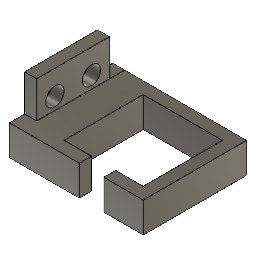
holder_R v6 (Autodesk Fusion 360 design; units mm, degrees)
Autodesk Fusion 360 part; units mm, degrees
sketch "Sketch1" plane through (0, 0, 0) normal (0, 0, 1) x (1, 0, 0)
  line L0 (0, 0) -> (13, 0)
  line L1 (13, 0) -> (13, 13)
  line L2 (13, 13) -> (0, 13)
  line L3 (0, 13) -> (0, 0)
  line L4 (-2, -2) -> (15, -2)
  line L5 (15, -2) -> (15, 15)
  line L6 (15, 15) -> (-2, 15)
  line L7 (-2, 15) -> (-2, -2)
  dimension "d1" = 13
  dimension "d2" = 13
  dimension "d3" = 2
  constraint horizontal L0
  constraint vertical L1
  constraint horizontal L2
  constraint vertical L3
  constraint coincident L0.start L3.end
  measures "d1" distance of L1.end L2.end
  measures "d2" distance of L0.end L1.end
extrude "Extrude1" add sketch "Sketch1" along normal blind 5
sketch "Sketch2" plane through (0, 0, 0) normal (0, 1, 0) x (-1, 0, 0)
  line L0 (-13, 0) -> (0, 0)
  line L1 (0, 0) -> (0, 5)
  line L2 (0, 5) -> (-13, 5)
  line L3 (-13, 5) -> (-13, 0)
  line L4 (-8.5, 5) -> (-4.5, 5)
  line L5 (-4.5, 5) -> (-4.5, 0)
  line L6 (-4.5, 0) -> (-8.5, 0)
  line L7 (-8.5, 0) -> (-8.5, 5)
  line L8 (-6.5, 0) -> (-6.5, 5)
  dimension "d6" = 4
  dimension "d7" = 90
  constraint horizontal L4
  constraint vertical L5
  constraint horizontal L6
  constraint vertical L7
  constraint coincident L0 L5.end
  constraint coincident L2 L4.start
  constraint midpoint L6 L8.start
  constraint midpoint L2 L8.end
  measures "d6" distance of L4.start L4.end
  measures "d7" angle of L4 L8
extrude "Extrude2" cut sketch "Sketch2" against normal blind 10 contours L0 L2 L4 L6 L7 L8 | L0 L2 L4 L5 L6 L8
extrude "Extrude3" add 1 faces at (-2, 9.3333, 1.6667) along direction (-1, 0, 0) blind 5
sketch "Sketch3" plane through (0, 0, 0) normal (0, 0, -1) x (1, 0, 0)
  line L0 (8.5, 2) -> (8.5, 0)
  line L1 (8.5, 0) -> (13, 0)
  line L2 (13, 0) -> (13, -13)
  line L3 (13, -13) -> (0, -13)
  line L4 (0, -13) -> (0, 0)
  line L5 (0, 0) -> (4.5, 0)
  line L6 (4.5, 0) -> (4.5, 2)
  line L7 (4.5, 2) -> (-7, 2)
  line L8 (-7, 2) -> (-7, -15)
  line L9 (-7, -15) -> (15, -15)
  line L10 (15, -15) -> (15, 2)
  line L11 (15, 2) -> (8.5, 2)
  line L12 (-7, 2) -> (-5, 2)
  line L13 (-5, 2) -> (-5, -15)
  line L14 (-5, -15) -> (-7, -15)
  line L15 (-7, -15) -> (-7, 2)
  dimension "d12" = 2
  constraint horizontal L12
  constraint vertical L13
  constraint horizontal L14
  constraint vertical L15
  constraint coincident L9 L13.end
  constraint coincident L7.end L8.start
  measures "d12" distance of L7.end L12.end
extrude "Extrude4" add sketch "Sketch3" along normal blind 6 contours L7 L8 L9 L12 L13 L14 L15
sketch "Sketch4" plane through (-5, 0, 0) normal (1, 0, 0) x (0, 1, 0)
  line L0 (15, 0) -> (-2, 0)
  line L1 (-2, 0) -> (-2, -6)
  line L2 (-2, -6) -> (15, -6)
  line L3 (15, -6) -> (15, 0)
  line L4 (-2, -2) -> (15, -2)
  circle A0 centre (3.5, -2) radius 1.5
  circle A1 centre (9.5, -2) radius 1.5
  line L5 (3.5, -2) -> (9.5, -2)
  line L6 (6.5, -2) -> (6.5, 0)
  dimension "d15" = 2
  dimension "d16" = 3
  dimension "d17" = 3
  dimension "d18" = 6
  dimension "d19" = 90
  constraint coincident L1 L4.start
  constraint coincident L3 L4.end
  constraint perpendicular L3 L4
  constraint coincident L4 A0.centre
  constraint coincident L4 A1.centre
  constraint coincident A0.centre L5.start
  constraint coincident A1.centre L5.end
  constraint midpoint L5 L6.start
  constraint midpoint L0 L6.end
  measures "d15" distance of L0 L4
  measures "d16" diameter of A0
  measures "d17" diameter of A1
  measures "d18" distance of A0.centre A1.centre
  measures "d19" angle of L0 L6
extrude "Extrude5" cut sketch "Sketch4" against normal blind 5 contours L4 A1 L5 | L4 A1 L5 | L4 A0 L5 | L4 A0 L5
mirror "Mirror1" about plane through (-2, 15, 5) normal (0, 0, 1) of bodies 1 merged
sketch "Sketch5" plane through (15, 0, 0) normal (1, 0, 0) x (0, 1, 0)
  line L0 (-2, 0) -> (15, 0)
  line L1 (15, 0) -> (15, 10)
  line L2 (15, 10) -> (-2, 10)
  line L3 (-2, 10) -> (-2, 0)
  line L4 (-15, 5) -> (21, 5)
  line L5 (21, 5) -> (21, -10.6123)
  line L6 (21, -10.6123) -> (-15, -10.6123)
  line L7 (-15, -10.6123) -> (-15, 5)
  constraint horizontal L4
  constraint vertical L5
  constraint horizontal L6
  constraint vertical L7
extrude "Extrude6" cut sketch "Sketch5" against normal blind 100 contours L0 L1 L3 L4 | L0 L1 L3 L4 L5 L6 L7
sketch "Sketch6" plane through (-5, 0, 0) normal (1, 0, 0) x (0, 1, 0)
  circle A0 centre (3.5, 12) radius 1.5
  circle A1 centre (9.5, 12) radius 1.5
  line L0 (-2, 10) -> (15, 10)
  line L1 (15, 10) -> (15, 16)
  line L2 (15, 16) -> (-2, 16)
  line L3 (-2, 16) -> (-2, 10)
  line L4 (-2, 16) -> (0.5, 16)
  line L5 (0.5, 16) -> (0.5, 10)
  line L6 (0.5, 10) -> (-2, 10)
  line L7 (-2, 10) -> (-2, 16)
  line L8 (15, 16) -> (12.5, 16)
  line L9 (12.5, 16) -> (12.5, 10)
  line L10 (12.5, 10) -> (15, 10)
  line L11 (15, 10) -> (15, 16)
  dimension "d26" = 3
  dimension "d27" = 3
  constraint horizontal L4
  constraint vertical L5
  constraint horizontal L6
  constraint vertical L7
  constraint coincident L0 L5.end
  constraint coincident L2.end L3.start
  constraint horizontal L8
  constraint vertical L9
  constraint horizontal L10
  constraint vertical L11
  constraint coincident L0 L9.end
  constraint coincident L1.end L2.start
  measures "d26" distance of A0.centre L5
  measures "d27" distance of A1.centre L9
extrude "Extrude7" cut sketch "Sketch6" against normal blind 6 contours L0 L2 L3 L4 L5 L6 L7 | L0 L1 L2 L8 L9 L10 L11
